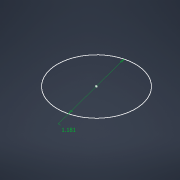
# Autodesk Inventor part: z axis-motor coupling
Saved by Autodesk Inventor 2021 (Build 250183000, 183)
## iProperties
Created: 2021-02-13
Part Number: z axis-motor coupling
Material: Generic
Document SubType Name: Modeling
Designer: ASUS
Density: 1 g/cm^3
Appearance: Flaked Satin - Blue
Author: ASUS
Autodesk Inventor part; units mm, degrees
ref_plane "YZ Plane" through (0, 0, 0) normal (1, 0, 0) x (0, 1, 0)
ref_plane "XZ Plane" through (0, 0, 0) normal (0, 1, 0) x (-1, 0, 0)
ref_plane "XY Plane" through (0, 0, 0) normal (0, 0, 1) x (1, 0, 0)
sketch "Sketch1" plane through (0, 0, 0) normal (0, 1, 0) x (-1, 0, 0)
  circle A0 centre (0, 0) radius 15
  circle A1 centre (0, 0) radius 3
  circle A2 centre (0, 10) radius 2
  circle A3 centre (-10, 0) radius 2
  circle A4 centre (0, -10) radius 2
  circle A5 centre (10, 0) radius 2
  dimension "d0" = 30
  dimension "d1" = 6
  dimension "d2" = 10
  dimension "d3" = 4
  dimension "d6" = 360
  constraints: 6 centre point, 2 coincident, 9 other
  measures "d0" diameter of A0
  measures "d1" diameter of A1
  measures "d2" distance of point (0, 0) A2.centre
  measures "d3" diameter of A2
extrude "Extrusion1" add sketch "Sketch1" along normal blind 3
sketch "Sketch2" plane through (0, 3, 0) normal (0, 1, 0) x (1, 0, 0)
  circle A0 centre (0, 0) radius 5.5
  circle A1 centre (0, 0) radius 3 projected
  dimension "d10" = 11
  constraints: 1 centre point, 1 coincident
  measures "d10" diameter of A0
extrude "Extrusion2" add sketch "Sketch2" along normal blind 15
chamfer "Chamfer1" distance 1 angle 45 2 edges at (15, 3, 0) (-5.5, 18, 0)
sketch "Sketch3" plane through (0, 0, 0) normal (0, 0, 1) x (1, 0, 0)
  circle A0 centre (0, 14) radius 1.5
  line L0 (-4.5, 18) -> (4.5, 18) projected
  point P0 (0, 0)
  dimension "d16" = 4
  dimension "d17" = 3
  constraints: 1 centre point
  measures "d16" distance from line of A0.centre L0
  measures "d17" diameter of A0
extrude "Extrusion3" cut sketch "Sketch3" along normal mid plane 15
body "Solid1"
